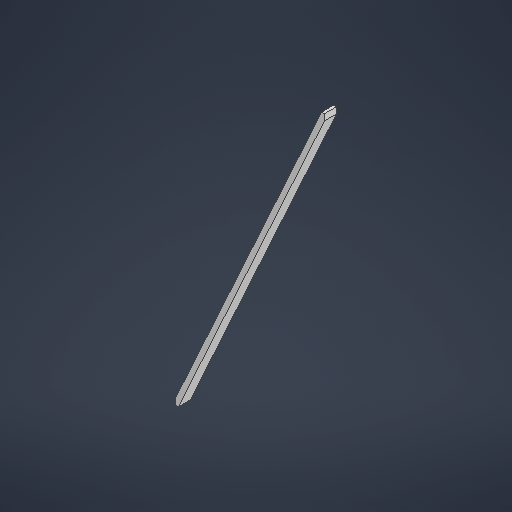
# Autodesk Inventor part: S_2x4x105.499
Saved by Autodesk Inventor 2026 (Build 300175000, 175)
## iProperties
Created: 2025-09-05
Part Number: S_2x4x105.499
Material: Generic
Document SubType Name: Modeling
Designer: trott
Density: 1 g/cm^3
Appearance: Default
Author: trott
Autodesk Inventor part; units mm, degrees
ref_plane "YZ Plane" through (0, 0, 0) normal (1, 0, 0) x (0, 1, 0)
ref_plane "XZ Plane" through (0, 0, 0) normal (0, 1, 0) x (-1, 0, 0)
ref_plane "XY Plane" through (0, 0, 0) normal (0, 0, 1) x (1, 0, 0)
sketch "Sketch1" plane through (0, 0, 0) normal (0, 0, 1) x (1, 0, 0)
  line L0 (-555.625, -1219.2) -> (555.625, -1219.2)
  line L1 (555.625, -1219.2) -> (555.625, 1219.2)
  line L2 (555.625, 1219.2) -> (-555.625, 1219.2)
  line L3 (-555.625, 1219.2) -> (-555.625, -1219.2)
  line L4 (-555.625, -1219.2) -> (555.625, 1219.2) construction
  line L5 (555.625, -1219.2) -> (-555.625, 1219.2) construction
  line L6 (555.625, 1219.2) -> (-555.625, -1219.2)
  line L7 (-538.2903, -1227.0999) -> (-572.9597, -1211.3001)
  line L8 (572.9597, 1211.3001) -> (538.2903, 1227.0999)
  line L9 (538.2903, 1227.0999) -> (-572.9597, -1211.3001)
  line L10 (-538.2903, -1227.0999) -> (572.9597, 1211.3001)
  point P0 (0, 0)
  point P1 (534.69, 1219.2)
  point P2 (-555.625, -1173.2627)
  point P3 (-534.69, -1219.2)
  point P4 (555.625, 1173.2627)
  dimension "d0" = 1111.25
  dimension "d1" = 2438.4
  dimension "d2" = 38.1
  dimension "d3" = 38.1
  constraints: 22 end point, 4 midpoint, 3 equal length, 3 perpendicular, 1 horizontal
  measures "d0" distance of L2.end L1.end
  measures "d1" distance of L0.end L1.end
  measures "d2" distance of L7.start L7.end
  measures "d3" distance of L8.start L8.end
extrude "Extrusion1" add sketch "Sketch1" along normal blind 88.9 contours L6 L1 L10 L0 | L3 L9 L2 L6
body "Solid1"
